pully 2GT-6mm 8mm v5 (Autodesk Fusion 360 design; units mm, degrees)
Autodesk Fusion 360 part; units mm, degrees
sketch "Sketch1" plane through (0, 0, 0) normal (0, 0, 1) x (1, 0, 0)
  circle A0 centre (0, 0) radius 12.5
  circle A1 centre (0, 0) radius 4
  dimension "d1" = 25
  dimension "d2" = 8
  constraint coincident A0.centre A1.centre
  measures "d1" diameter of A0
  measures "d2" diameter of A1
extrude "Extrude1" add sketch "Sketch1" along normal blind 7.6
sketch "Sketch2" plane through (0, 0, 7.6) normal (0, 0, 1) x (-1, 0, 0)
  circle A0 centre (0, 0) radius 4
  circle A1 centre (0, 0) radius 12.5
  circle A2 centre (0, 0) radius 18.85
  circle A3 centre (0, 0) radius 21.8
  dimension "d5" = 37.7
  dimension "d11" = 43.6
  constraint coincident A0.centre A1.centre
  constraint concentric A2 A3
  measures "d5" diameter of A2
  measures "d11" diameter of A3
extrude "Extrude2" add sketch "Sketch2" along normal blind 7 contours A1 | A2
sketch "Sketch3" plane through (0, 0, 14.6) normal (0, 0, 1) x (-1, 0, 0)
  circle A0 centre (0, 0) radius 4
  circle A1 centre (0, 0) radius 18.85
  circle A2 centre (0, 0) radius 21.8
  dimension "d8" = 43.6
  constraint coincident A0.centre A1.centre
  measures "d8" diameter of A2
extrude "Extrude3" add sketch "Sketch3" along normal blind 1.5 contours A1 | A2
extrude "Extrude4" add sketch "Sketch2" against normal blind 1.5 contours A2 | A3
